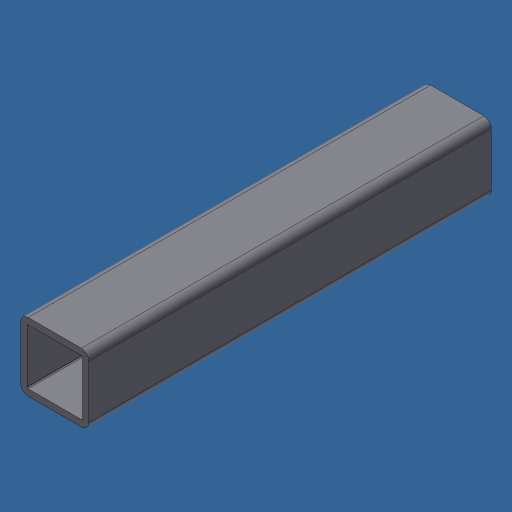
# Autodesk Inventor part: TUBE
Saved by Autodesk Inventor 2024.3 (Build 283343000, 343)
## iProperties
ILogicPurgeVersion: 0.0.0.0
OnSaveVersion: 2.2.20.20
RuleStatus: InUse
Category: _
Manager: _
Created: 2023-11-08
Part Number: TUBE
Checked By: 0002334344
Engr Approved By: R
User Status: Work In Process
Material: Steel, MS
Description: TEMPLATE,TUBING
Document SubType Name: Modeling
Mfg Approved By: Stephen.Oerton
Designer: Raamprakash.Soundaran
Mass: 2006.79 g
Surface Area: 1089.22 cm^2
Volume: 255.316 cm^3
Density: 7.86 g/cm^3
Appearance: Metal-Steel
CN_MASS: 2.01
PTC_WM_ITERATION: 1
PTC_WM_ORGANIZATION_ID: CLWC
PTC_WM_LIFECYCLE: CLWC_CAD_LC
CL_runCount: 0
Length: 0.19" WALL X 2" X 2" X 300.0 mm Lg
ModelCat: Tube
FIRST_DESCRIPTION: _
SECOND_DESCRIPTION: _
THIRD_DESCRIPTION: _
CN_SERVICEABLE: _
Subject: _
Author: Raamprakash.Soundaran
Keywords: -
Revision Number: A
Autodesk Inventor part; units mm, degrees
ref_plane "YZ Plane" through (0, 0, 0) normal (1, 0, 0) x (0, 1, 0)
ref_plane "XZ Plane" through (0, 0, 0) normal (0, 1, 0) x (-1, 0, 0)
ref_plane "XY Plane" through (0, 0, 0) normal (0, 0, 1) x (1, 0, 0)
sketch "Sketch1" plane through (0, 0, 0) normal (0, 0, 1) x (1, 0, 0)
  line L0 (-25.4, 25.4) -> (25.4, 25.4)
  line L1 (25.4, 25.4) -> (25.4, -25.4)
  line L2 (25.4, -25.4) -> (-25.4, -25.4)
  line L3 (-25.4, -25.4) -> (-25.4, 25.4)
  line L4 (0, 0) -> (0, -25.4) construction
  line L5 (-53.34, 0) -> (53.34, 0) construction
  dimension "d10" = 25.4
  dimension "RotateAngle" = 90
  constraints: 10 end point, 2 parallel, 1 horizontal alignment, 1 midpoint, 1 perpendicular, 1 vertical alignment, 1 other
  measures "d10" distance from line of L4.start L0
  measures "RotateAngle" angle of L4 L5
extrude "Extrusion1" add sketch "Sketch1" along normal mid plane 300
fillet "Fillet1" radius 5.5563 4 edges at (-25.4, 25.4, 0) (-25.4, -25.4, 0) (25.4, 25.4, 0) (25.4, -25.4, 0)
shell "Shell1" thickness 4.7625 removed faces 2 at (-8.4667, -6.6146, 150) at (-8.4667, -6.6146, -150)
feature "TaperEdge1-YZ" [suppressed]
feature "TaperEdge2-YZ" [suppressed]
feature "TaperEdge1-XZ" [suppressed]
feature "TaperEdge2-XZ" [suppressed]
sketch "Sketch4" plane through (0, -63.5, 762) normal (1, 0, 0) x (0, 0, -1)
  line L0 (254.5, 63.5) -> (534.5, 63.5) construction
  line L1 (254.5, 26) -> (534.5, 26)
  line L2 (534.5, 101) -> (254.5, 101)
  arc A0 (254.5, 101) -> (254.5, 26) centre (254.5, 63.5) ccw
  arc A1 (534.5, 26) -> (534.5, 101) centre (534.5, 63.5) ccw
  line L3 (989.5, 63.5) -> (1269.5, 63.5) construction
  line L4 (989.5, 26) -> (1269.5, 26)
  line L5 (1269.5, 101) -> (989.5, 101)
  arc A2 (989.5, 101) -> (989.5, 26) centre (989.5, 63.5) ccw
  arc A3 (1269.5, 26) -> (1269.5, 101) centre (1269.5, 63.5) ccw
  point P0 (762, 63.5)
  point P1 (394.5, 63.5)
  point P2 (1129.5, 63.5)
  dimension "d24" = 280
  dimension "d25" = 75
  dimension "d27" = 1015
  dimension "d28" = 507.5
  constraints: 16 end point, 8 point on circle, 8 tangent, 4 centre point, 2 midpoint, 2 parallel, 2 point on line, 1 collinear, 1 equal radius, 1 horizontal, 1 horizontal alignment
  measures "d24" distance of L0.start L0.end
  measures "d25" distance between parallel lines of L1 L2
  measures "d27" distance of L3.end L0.start
  measures "d28" distance of point (762, 63.5) L0.start
extrude "ForkSlots" [suppressed]
